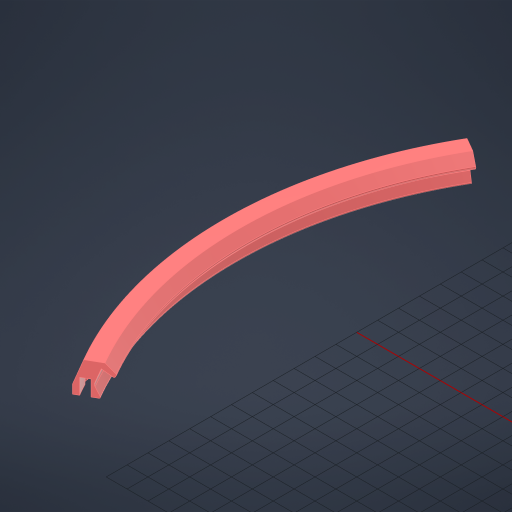
# Autodesk Inventor part: LED-Ring_Element_v2
Saved by Autodesk Inventor 2023.2 (Build 272271030, 271C)
## iProperties
Created: 2023-02-18
Part Number: LED-Ring_Element_v2
Material: Generisch
Document SubType Name: Modeling
Designer: Stefan
Mass: 162.723 g
Surface Area: 538.591 cm^2
Volume: 162.723 cm^3
Density: 1 g/cm^3
Appearance: Glatt - Rot
Author: Stefan
Autodesk Inventor part; units mm, degrees
ref_plane "YZ Plane" through (0, 0, 0) normal (1, 0, 0) x (0, 1, 0)
ref_plane "XZ Plane" through (0, 0, 0) normal (0, 1, 0) x (-1, 0, 0)
ref_plane "XY Plane" through (0, 0, 0) normal (0, 0, 1) x (1, 0, 0)
sketch "Skizze1" plane through (0, 0, 0) normal (0, 0, 1) x (1, 0, 0)
  arc A0 (-346.4361, 139.3117) -> (-345.0142, 139.6704) centre (-345.8915, 140.1504) ccw
  line L0 (-344.2531, 141.0614) -> (-345.0142, 139.6704)
  arc A1 (-344.2531, 141.0614) -> (-344.4232, 142.2486) centre (-345.1303, 141.5415) ccw
  line L1 (-352.1746, 150) -> (-344.4232, 142.2486)
  line L2 (-367.1746, 150) -> (-352.1746, 150)
  line L3 (-375, 128.5) -> (-367.1746, 150)
  line L4 (-375, 120) -> (-375, 128.5)
  line L5 (-356.3704, 120) -> (-375, 120)
  line L6 (0, 0) -> (-360, 0) construction
  line L7 (-356.9218, 139.1504) -> (-345, 0) construction
  line L8 (-356.9218, 139.1504) -> (0, 139.1504) construction
  line L9 (0, 139.1504) -> (0, 0) construction
  line L10 (-360, 130.6932) -> (-360, 0) construction
  line L11 (0, 0) -> (-225, 0) construction
  line L12 (-225, 0) -> (-225, 50) construction
  line L13 (-225, 50) -> (0, 50) construction
  line L14 (0, 50) -> (0, 0) construction
  line L15 (-346.4361, 139.3117) -> (-354.8697, 144.7886)
  line L16 (-360, 130.6932) -> (-355.4722, 121.4395)
  arc A2 (-356.3704, 120) -> (-355.4722, 121.4395) centre (-356.3704, 121) ccw
  line L17 (-225, 0) -> (-345, 0) construction
  line L18 (-345, 0) -> (-345, 35) construction
  line L19 (-345, 35) -> (-225, 35) construction
  line L20 (-225, 35) -> (-225, 0) construction
  line L21 (-354.8697, 144.7886) -> (-360, 130.6932)
  line L22 (-356.9218, 139.1504) -> (0, 9.2415) construction
  line L23 (-344.2531, 141.0614) -> (-355.4932, 120.52) construction
  line L24 (-368.25, 135) -> (-363.75, 135) construction
  line L25 (-363.75, 135) -> (-363.75, 141) construction
  line L26 (-363.75, 141) -> (-368.25, 141) construction
  line L27 (-368.25, 141) -> (-368.25, 135) construction
  line L28 (-367.6, 135) -> (-364.4, 135) construction
  line L29 (-364.4, 135) -> (-364.4, 129) construction
  line L30 (-364.4, 129) -> (-367.6, 129) construction
  line L31 (-367.6, 129) -> (-367.6, 135) construction
  line L32 (-369, 129) -> (-363, 129) construction
  line L33 (-363, 129) -> (-363, 126) construction
  line L34 (-363, 126) -> (-369, 126) construction
  line L35 (-369, 126) -> (-369, 129) construction
  arc A3 (-359.3455, 132.4913) -> (-359.159, 128.9744) centre (-355.1169, 130.9522) ccw
  line L36 (-362, 120) -> (-370, 120)
  line L37 (-370, 120) -> (-370, 135)
  line L38 (-370, 135) -> (-362, 135)
  line L39 (-362, 135) -> (-362, 120)
  line L40 (-370, 135) -> (-362, 135)
  line L41 (-362, 135) -> (-362, 126)
  line L42 (-362, 126) -> (-370, 126)
  line L43 (-370, 126) -> (-370, 135)
  line L44 (-360, 130.6932) -> (-360, 120)
  point P0 (-366, 129)
  point P1 (-366, 135)
  dimension "d1" = 30
  dimension "d5" = 1
  dimension "d9" = 135
  dimension "d14" = 8.5
  dimension "d18" = 360
  dimension "d25" = 50
  dimension "d26" = 225
  dimension "d31" = 15
  dimension "d40" = 3.5
  dimension "d41" = 120
  dimension "d42" = 35
  dimension "d43" = 1
  dimension "d47" = 6
  dimension "d50" = 65.103
  dimension "d54" = 15
  dimension "d59" = 12
  dimension "d60" = 160
  dimension "d66" = 15
  dimension "d70" = 4.5
  dimension "d71" = 6
  dimension "d73" = 3.2
  dimension "d74" = 3
  dimension "d75" = 6
  dimension "d76" = 6
  dimension "d77" = 6
  dimension "d79" = 4.5
  dimension "d80" = 15
  dimension "d81" = 2
  dimension "d82" = 8
  dimension "d83" = 120
  constraints: 90 end point, 15 parallel, 11 point on line, 10 horizontal, 10 tangent, 9 point on circle, 8 perpendicular, 5 midpoint, 4 centre point, 2 vertical, 1 collinear, 1 equal radius, 4 other
  measures "d1" distance between parallel lines of L5 L2
  measures "d5" radius of A1
  measures "d9" angle of L1 L2
  measures "d14" distance of L4.start L3.start
  measures "d18" distance of L6.end L6.start
  measures "d25" distance of L11.end L12.end
  measures "d26" distance of L12.end L13.end
  measures "d31" distance of L2.start L1.start
  measures "d40" distance from line of L15.start L1
  measures "d41" distance of L18.end L19.end
  measures "d42" distance of L17.end L18.end
  measures "d43" radius of A2
  measures "d47" distance of L15.end L8.start
  measures "d54" distance of L10.start L15.end
  measures "d59" angle of L1 L15
  measures "d60" angle of L10 L21
  measures "d66" distance between parallel lines of L10 L4
  measures "d70" distance between parallel lines of L25 L27
  measures "d71" distance between parallel lines of L24 L26
  measures "d73" distance between parallel lines of L29 L31
  measures "d74" distance of L34.end L32.start
  measures "d75" distance of L33.end L34.end
  measures "d76" distance between parallel lines of L28 L30
  measures "d77" distance between parallel lines of L5 L34
  measures "d79" radius of A3
  measures "d80" distance between parallel lines of L5 L38
  measures "d81" distance from line of L39 L10.start
  measures "d82" distance between parallel lines of L39 L37
  measures "d83" distance between parallel lines of L5 L6
revolve "Umdrehung1" add sketch "Skizze1" angle 60 mid plane about axis through (0, 139.1504, 0) along (0, -1, 0) contours L15 L21 L44 L5 L39 L38 L37 L4 L3 L2 L1 A1 L0 A0 | A3 L16 L21 | L16 A2 L5 L44
revolve "Umdrehung2" add sketch "Skizze1" angle 30 mid plane about axis through (0, 139.1504, 0) along (0, -1, 0) contours L42 L37 L38 L39
sketch "Skizze2" plane through (-320.4294, 135, -185) normal (0, -1, 0) x (0.866, 0, 0.5)
  arc A0 (185, 320.4294) -> (0, 0) centre (370, 0) ccw projected
  arc A1 (189, 313.5012) -> (8, 0) centre (370, 0) ccw projected
  line L0 (108.3705, 261.6295) -> (114.0273, 255.9727) projected
  arc A2 (108.3705, 261.6295) -> (12.6074, 95.763) centre (370, 0) ccw projected
  line L1 (20.3349, 93.6925) -> (12.6074, 95.763) projected
  arc A3 (114.0273, 255.9727) -> (20.3349, 93.6925) centre (370, 0) ccw projected
  line L2 (8, 0) -> (0, 0) projected
  line L3 (185, 320.4294) -> (189, 313.5012) projected
  arc A4 (187, 316.9653) -> (4, 0) centre (370, 0) ccw construction
  circle A5 centre (4.3484, 15.9647) radius 2.25
  circle A6 centre (12.6757, 79.2169) radius 2.25
  circle A7 centre (122.734, 269.8435) radius 2.25
  circle A8 centre (173.3483, 308.6813) radius 2.25
  line L4 (4.3484, 15.9647) -> (370, 0) construction
  line L5 (370, 0) -> (12.6757, 79.2169) construction
  line L6 (122.734, 269.8435) -> (370, 0) construction
  line L7 (173.3483, 308.6813) -> (370, 0) construction
  line L8 (4, 0) -> (370, 0) construction
  line L9 (187, 316.9653) -> (370, 0) construction
  circle A9 centre (173.3483, 308.6813) radius 5
  circle A10 centre (122.734, 269.8435) radius 5
  circle A11 centre (12.6757, 79.2169) radius 5
  circle A12 centre (4.3484, 15.9647) radius 5
  dimension "d85" = 2.5
  dimension "d86" = 10
  dimension "d87" = 2.5
  dimension "d88" = 10
  dimension "d89" = 4.5
  dimension "d97" = 10
  constraints: 12 end point, 9 centre point, 6 equal radius, 6 point on circle, 5 coincident, 2 midpoint, 1 horizontal
  measures "d85" angle of L4 L8
  measures "d86" angle of L5 L4
  measures "d87" angle of L9 L7
  measures "d88" angle of L6 L7
  measures "d89" diameter of A5
  measures "d97" diameter of A12
hole "Bohrung1" at (-324.646, 135, -169) at (-349.0604, 135, -110.0583) at (-349.0604, 135, 110.0583) at (-324.646, 135, 169) direction (0, 1, 0) diameter 4.5 depth 6
extrude "Extrusion1" cut sketch "Skizze2" along normal through all contours A10 A0 | A0 A10 A1 | A11 A1 A0 | A0 A11 | A1 A10 | A11 A1 | A9 A0 | A0 A9 A1 | A12 A1 A0 | A0 A12 | A1 A9 | A12 A1 | A5 | A6 | A7 | A8
